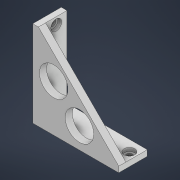
# Autodesk Inventor part: Buttons_Mount_v1
Saved by Autodesk Inventor 2022 (Build 260153000, 153)
## iProperties
Created: 2022-01-30
Part Number: Buttons_Mount_v1
Material: Generisch
Document SubType Name: Modeling
Designer: Martin
Density: 1 g/cm^3
Appearance: Vorgabe
Author: Martin
Autodesk Inventor part; units mm, degrees
ref_plane "YZ Plane" through (0, 0, 0) normal (1, 0, 0) x (0, 1, 0)
ref_plane "XZ Plane" through (0, 0, 0) normal (0, 1, 0) x (-1, 0, 0)
ref_plane "XY Plane" through (0, 0, 0) normal (0, 0, 1) x (1, 0, 0)
sketch "Skizze1" plane through (0, 0, 0) normal (0, 0, 1) x (1, 0, 0)
  line L0 (0, 0) -> (45, 0)
  line L1 (45, 0) -> (0, 45)
  line L2 (0, 45) -> (0, 0)
  dimension "d0" = 45
  dimension "d1" = 45
  constraints: 6 end point, 1 horizontal, 1 perpendicular
  measures "d0" distance of L0.start L0.end
  measures "d1" distance of L1.end L0.start
extrude "Extrusion1" add sketch "Skizze1" along normal blind 4
sketch "Skizze4" plane through (0, 0, 4) normal (0, 0, 1) x (1, 0, 0)
  line L0 (45, 0) -> (0, 45) projected
  line L1 (45, 0) -> (45, -3.2)
  line L2 (45, -3.2) -> (-3.2, -3.2)
  line L3 (-3.2, -3.2) -> (-3.2, 45)
  line L4 (-3.2, 45) -> (0, 45)
  line L5 (0, 0) -> (45, 0) projected
  line L6 (0, 45) -> (0, 0) projected
  dimension "d20" = 3.2
  dimension "d21" = 3.2
  constraints: 8 end point, 3 perpendicular, 1 vertical
  measures "d20" distance of L0.start L1.end
  measures "d21" distance of L3.end L0.end
extrude "Extrusion3" add sketch "Skizze4" against normal blind 16 contours L1 L2 L3 L4 L6 L5
sketch "Skizze2" plane through (0, 0, 4) normal (0, 0, 1) x (1, 0, 0)
  line L0 (45, 0) -> (0, 45) projected
  point P0 (0, 0)
  point P1 (8.565, 23)
  point P2 (23, 8.565)
  dimension "d11" = 9.5
  dimension "d12" = 9.5
  dimension "d14" = 22
  dimension "d15" = 22
  measures "d11" distance from line of point (8.565, 23) L0
  measures "d12" distance from line of L0 point (23, 8.565)
  measures "d14" vertical distance of L0.end point (8.565, 23)
  measures "d15" horizontal distance of L0.start point (23, 8.565)
hole "Bohrung1" at (8.565, 23, 4) at (23, 8.565, 4) direction (0, 0, -1) diameter 16 end through all
sketch "Skizze5" plane through (0, 0, 0) normal (0, 1, 0) x (1, 0, 0)
  line L0 (45, 0) -> (45, 12) projected
  line L1 (45, 0) -> (0, 0) projected
  point P0 (41, 6)
  dimension "d31" = 4
  dimension "d32" = 6
  measures "d31" distance from line of point (41, 6) L0
  measures "d32" distance from line of point (41, 6) L1
hole "Bohrung2" at (41, 0, -6) direction (0, -1, 0) diameter 3.5 end through all counterbore diameter 6 counterbore depth 2
sketch "Skizze6" plane through (0, 0, 0) normal (1, 0, 0) x (0, 0, -1)
  line L0 (0, 0) -> (0, 45) projected
  line L1 (0, 45) -> (12, 45) projected
  point P0 (6, 41)
  dimension "d40" = 6
  dimension "d41" = 4
  measures "d40" distance from line of point (6, 41) L0
  measures "d41" distance from line of L1 point (6, 41)
hole "Bohrung3" at (0, 41, -6) direction (-1, 0, 0) diameter 3.5 end through all counterbore diameter 6 counterbore depth 2
equation "\"d0\" = d1"
equation "\"d21\" = d20"
equation "\"d12\" = d11"
equation "\"d15\" = d14"
